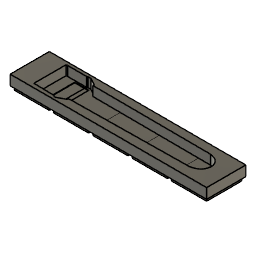
bed scraper gridfinity module (Autodesk Fusion 360 design; units mm, degrees)
Autodesk Fusion 360 part; units mm, degrees
sketch "Sketch1" plane through (0, 0, 0) normal (0, 0, 1) x (1, 0, 0)
  line L0 (20.75, -20.75) -> (-20.75, -20.75)
  line L1 (-20.75, -20.75) -> (-20.75, 20.75)
  line L2 (-20.75, 20.75) -> (20.75, 20.75)
  line L3 (20.75, 20.75) -> (20.75, -20.75)
  line L4 (20.75, -20.75) -> (-20.75, 20.75) construction
  line L5 (-20.75, -20.75) -> (20.75, 20.75) construction
  dimension "d1" = 41.5
  dimension "d2" = 41.5
  constraint horizontal L0
  constraint perpendicular L0 L1
  constraint parallel L0 L2
  constraint parallel L1 L3
  constraint coincident L4 origin
  constraint coincident L5 origin
  measures "d1" distance of L1.end L2.end
  measures "d2" distance of L0.end L1.end
extrude "Extrude1" add sketch "Sketch1" along normal blind 7 makes body 1
sketch "Sketch2" plane through (0, -20.75, 0) normal (0, -1, 0) x (1, 0, 0)
  line L0 (-20.75, 0) -> (20.75, 0)
  line L1 (20.75, 0) -> (20.75, 7)
  line L2 (20.75, 7) -> (-20.75, 7)
  line L3 (-20.75, 7) -> (-20.75, 0)
  line L4 (20.75, 0) -> (17.8, 0) construction
  line L5 (17.8, 0) -> (18.6, 0) construction
  line L6 (17.8, 0) -> (18.6, 0.8)
  line L7 (18.6, 0.8) -> (18.6, 2.6)
  line L8 (18.6, 2.6) -> (20.75, 4.75)
  line L9 (-17.8, 0) -> (-18.6, 0.8)
  line L10 (-18.6, 0.8) -> (-18.6, 2.6)
  line L11 (-18.6, 2.6) -> (-20.75, 4.75)
  constraint coincident L0.end L1.start
  constraint perpendicular L1 L4
  constraint parallel L4 L5
  constraint perpendicular L4 L7
  constraint coincident L1 L8.end
  constraint coincident L3 L11.end
sketch "Sketch3" plane through (20.75, 0, 0) normal (1, 0, 0) x (0, 1, 0)
  line L0 (-20.75, 0) -> (20.75, 0)
  line L1 (20.75, 0) -> (20.75, 7)
  line L2 (20.75, 7) -> (-20.75, 7)
  line L3 (-20.75, 7) -> (-20.75, 0)
  line L4 (-17.8, 0) -> (-18.6, 0.8)
  line L5 (-18.6, 0.8) -> (-18.6, 2.6)
  line L6 (-18.6, 2.6) -> (-20.75, 4.75)
  line L7 (18.6, 0.8) -> (18.6, 2.6)
  line L8 (18.6, 2.6) -> (20.75, 4.75)
  line L9 (17.8, 0) -> (18.6, 0.8)
  constraint coincident L3 L6.end
  constraint perpendicular L0 L7
  constraint coincident L1 L8.end
extrude "Extrude2" cut sketch "Sketch3" along normal mid plane 100 contours L0 L3 L4 L5 L6 | L0 L1 L7 L8 L9 bodies 1
extrude "Extrude3" cut sketch "Sketch2" along normal mid plane 100 contours L0 L3 L9 L10 L11 | L0 L1 L6 L7 L8 bodies 1
move_body "Move1" bodies 1 to x (1, 0, 0) y (0, 1, 0) z (0, 0, 1) at (0, 7.0711, -7.0711)
copy_body "CopyPasteBodies1" bodies 1 makes body 2
move_body "Move2" bodies 2 to x (1, 0, 0) y (0, 1, 0) z (0, 0, 1) at (41.5, 0, 0)
copy_body "CopyPasteBodies2" bodies 2 makes body 3
move_body "Move3" bodies 3 to x (1, 0, 0) y (0, 1, 0) z (0, 0, 1) at (41.5, 0, 0)
copy_body "CopyPasteBodies3" bodies 3 makes body 4
move_body "Move4" bodies 4 to x (1, 0, 0) y (0, 1, 0) z (0, 0, 1) at (41.5, 0, 0)
copy_body "CopyPasteBodies4" bodies 4 makes body 5
move_body "Move5" bodies 5 to x (1, 0, 0) y (0, 1, 0) z (0, 0, 1) at (41.5, 0, 0)
combine "Combine1" operation add target body 1 tool bodies 4 5 3 2
move_body "Move6" bodies 1 to x (1, 0, 0) y (0, 1, 0) z (0, 0, 1) at (0, -21.59, 0)
move_body "Move7" bodies 1 to x (1, 0, 0) y (0, 1, 0) z (0, 0, 1) at (-50.8, 0, 0)
sketch "Sketch4" plane through (0, 0, -0.0711) normal (0, 0, 1) x (-1, 0, 0)
  line L0 (-135.95, -6.2311) -> (71.55, -6.2311)
  line L1 (71.55, -6.2311) -> (71.55, 35.2689)
  line L2 (71.55, 35.2689) -> (-135.95, 35.2689)
  line L3 (-135.95, 35.2689) -> (-135.95, -6.2311)
  line L4 (49, -3) -> (29, -3)
  line L5 (29, -3) -> (28, -3.5)
  line L6 (28, -3.5) -> (25, -3.5)
  line L7 (25, -3.5) -> (17.5, 0.5)
  line L8 (17.5, 0.5) -> (17.5, 2)
  line L9 (17.5, 2) -> (-107.4999, 2.694)
  spline S0 degree 5 poles (-107.4999, 2.694) (-107.5377, 2.6996) (-107.6224, 2.7132) (-107.7771, 2.7406) (-108.0391, 2.7914) (-108.4586, 2.8788) (-108.9665, 2.9906) (-109.553, 3.1272) (-110.2001, 3.2888) (-110.8844, 3.4752) (-111.5802, 3.6861) (-112.2621, 3.9209) (-112.9086, 4.1785) (-113.5044, 4.457) (-114.0439, 4.7543) (-114.5289, 5.0673) (-114.9659, 5.3933) (-115.3638, 5.7293) (-115.7318, 6.0731) (-116.0766, 6.4227) (-116.4024, 6.7772) (-116.6494, 7.0643) (-116.8275, 7.2814) (-116.943, 7.427) (-117, 7.5) knots 0 0 0 0 0 0 0.05 0.1 0.15 0.2 0.25 0.3 0.35 0.4 0.45 0.5 0.55 0.6 0.65 0.7 0.75 0.8 0.85 0.9 0.95 1 1 1 1 1 1
  spline S1 degree 5 poles (-117, 7.5) (-117.0188, 7.5092) (-117.0564, 7.532) (-117.1123, 7.5793) (-117.186, 7.669) (-117.2835, 7.8311) (-117.4084, 8.061) (-117.5856, 8.3788) (-117.8277, 8.7933) (-118.1204, 9.2905) (-118.4329, 9.8427) (-118.7279, 10.419) (-118.9706, 10.9934) (-119.1407, 11.5563) (-119.2363, 12.118) (-119.2655, 12.6987) (-119.2412, 13.3224) (-119.1752, 14.0093) (-119.071, 14.7675) (-118.9241, 15.593) (-118.724, 16.4731) (-118.4565, 17.3893) (-118.1056, 18.3198) (-117.6551, 19.2424) (-117.0913, 20.1373) (-116.4042, 20.9895) (-115.587, 21.7876) (-114.6352, 22.5237) (-113.5466, 23.1925) (-112.3203, 23.7909) (-110.9565, 24.3173) (-109.7558, 24.6804) (-108.7941, 24.9203) (-108.1257, 25.0657) (-107.7847, 25.1349) knots 0 0 0 0 0 0 0.033333 0.066667 0.1 0.133333 0.166667 0.2 0.233333 0.266667 0.3 0.333333 0.366667 0.4 0.433333 0.466667 0.5 0.533333 0.566667 0.6 0.633333 0.666667 0.7 0.733333 0.766667 0.8 0.833333 0.866667 0.9 0.933333 0.966667 1 1 1 1 1 1
  line L10 (-107.7847, 25.1349) -> (17.7875, 26.8161)
  line L11 (17.7875, 26.8161) -> (18.6921, 28.4126)
  line L12 (18.6921, 28.4126) -> (26.2768, 32.4251)
  line L13 (26.2768, 32.4251) -> (27.6742, 32.3957)
  line L14 (27.6742, 32.3957) -> (28.9778, 31.5395)
  line L15 (28.9778, 31.5395) -> (50.5586, 31.0849)
  line L16 (50.5586, 31.0849) -> (50.5586, -2.9257)
  line L17 (49, -3) -> (50.5586, -2.9257)
  line L18 (25.2438, -1.5) -> (40, -1.5)
  line L19 (40, -1.5) -> (40, 27)
  line L20 (40, 27) -> (25, 27)
  line L21 (25, 27) -> (25.2438, -1.5)
  point P0 (-109, 3)
  point P1 (-112.9229, 4.1954)
  point P2 (-115.4833, 5.8456)
  point P3 (-117.2, 7.7)
  point P4 (-117.6, 8.4)
  point P5 (-118.8673, 10.7685)
  point P6 (-119.2147, 13.547)
  point P7 (-117.6991, 19.1042)
  constraint horizontal L4
  constraint parallel L4 L6
  constraint perpendicular L6 L8
  constraint parallel L13 L15
  constraint vertical L16
  constraint parallel L0 L18
  constraint perpendicular L0 L19
  constraint perpendicular L19 L20
move_body "Move8" bodies 1 to x (1, 0, 0) y (0, 1, 0) z (0, 0, 1) at (0, 0, 1.5)
sketch "Sketch5" plane through (0, 0, 1.4289) normal (0, 0, 1) x (-1, 0, 0)
  line L0 (-135.95, -6.2311) -> (71.55, -6.2311)
  line L1 (71.55, -6.2311) -> (71.55, 35.2689)
  line L2 (71.55, 35.2689) -> (-135.95, 35.2689)
  line L3 (-135.95, 35.2689) -> (-135.95, -6.2311)
  line L4 (71.55, -6.2311) -> (-135.95, -6.2311)
  line L5 (-135.95, -6.2311) -> (-135.95, 35.2689)
  line L6 (-135.95, 35.2689) -> (71.55, 35.2689)
  line L7 (71.55, 35.2689) -> (71.55, -6.2311)
  constraint horizontal L4
  constraint vertical L5
  constraint horizontal L6
  constraint vertical L7
  constraint coincident L2.end L3.start
  constraint coincident L0.end L1.start
extrude "Extrude4" add sketch "Sketch5" along normal blind 8.5 bodies 1
move_body "Move9" bodies 1 to x (1, 0, 0) y (0, 1, 0) z (0, 0, 1) at (0, 0, -10)
extrude "Extrude5" cut sketch "Sketch4" against normal blind 10.5 contours L18 L19 L20 L21 bodies 1
extrude "Extrude6" cut sketch "Sketch4" against normal blind 10 contours L4 L5 L6 L7 L8 L9 S0 S1 L10 L11 L12 L13 L14 L15 L16 L17 bodies 1
